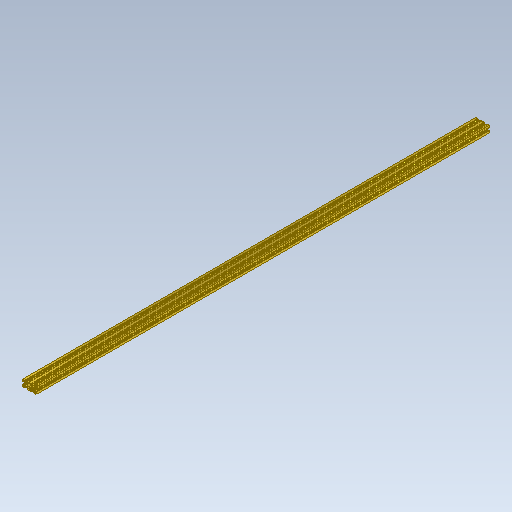
# Autodesk Inventor part: Perfil 30×60 6 rasgos_AST03006006
Saved by Autodesk Inventor 2025.2 (Build 292293000, 293)
## iProperties
Created: 2025-04-06
Part Number: Perfil 30×60 6 rasgos_AST03006006
Material: Ouro
Document SubType Name: Modeling
Designer: Gustavo Sousa
Density: 19.3 g/cm^3
Appearance: Metal quente 2400F
Author: Gustavo Sousa
Autodesk Inventor part; units mm, degrees
ref_plane "YZ Plane" through (0, 0, 0) normal (1, 0, 0) x (0, 1, 0)
ref_plane "XZ Plane" through (0, 0, 0) normal (0, 1, 0) x (-1, 0, 0)
ref_plane "XY Plane" through (0, 0, 0) normal (0, 0, 1) x (1, 0, 0)
sketch "Esboço1" plane through (0, 0, 0) normal (0, 0, 1) x (1, 0, 0)
  line L0 (-30, 15) -> (30, 15) construction
  circle A0 centre (-15, 0) radius 5 construction
  line L1 (-15, 0) -> (0, 15) construction
  line L2 (-22, 7) -> (-8, 7) construction
  line L3 (-19.1, 15) -> (-10.9, 15) construction
  line L4 (-30, 15) -> (-15, 15) construction
  line L5 (-22, 7) -> (-22, 0) construction
  line L6 (-30, 15) -> (-30, -15) construction
  line L7 (-19.1, 15) -> (-19.6, 15) construction
  line L8 (-19.6, 15) -> (-19.6, 14.5)
  line L9 (-19.6, 14.5) -> (-19.1, 14.5)
  line L10 (-19.1, 14.5) -> (-19.1, 15) construction
  line L11 (-19.1, 15) -> (-19.1, 12.8) construction
  line L12 (-19.1, 12.8) -> (-23.15, 12.8) construction
  line L13 (-19.1, 14.5) -> (-19.1, 12.8)
  line L14 (-22, 7) -> (-15, 0) construction
  line L15 (-22, 7) -> (-30, 15) construction
  arc A1 (-29.5, 15) -> (-30, 14.5) centre (-29.5, 14.5) ccw construction
  arc A2 (-29.5, 15) -> (-29.8536, 14.8536) centre (-29.5, 14.5) ccw
  line L16 (-29.5, 15) -> (-19.6, 15)
  line L17 (-23.15, 9.7056) -> (-20.4444, 7) construction
  line L18 (-23.15, 12.8) -> (-23.15, 9.7056) construction
  line L19 (-20.4444, 7) -> (-15, 7) construction
  circle A3 centre (-26.5, 11.5) radius 2.25 construction
  line L20 (-10.9, 15) -> (-10.4, 15) construction
  line L21 (-10.4, 15) -> (-10.4, 14.5)
  line L22 (-10.4, 14.5) -> (-10.9, 14.5)
  line L23 (-10.9, 14.5) -> (-10.9, 15) construction
  line L24 (-10.4, 15) -> (0, 15)
  line L25 (-10.9, 15) -> (-10.9, 12.8) construction
  line L26 (-10.9, 12.8) -> (-6.85, 12.8) construction
  line L27 (-10.9, 14.5) -> (-10.9, 12.8)
  line L28 (-9.5556, 7) -> (-6.85, 9.7056) construction
  line L29 (-6.85, 12.8) -> (-6.85, 9.7056) construction
  line L30 (-9.5556, 7) -> (-15, 7) construction
  line L31 (-8, 7) -> (-8, 0) construction
  line L32 (-22, 0) -> (-20, 0)
  line L33 (-10, 0) -> (-8, 0)
  line L34 (-4.65, 8.7944) -> (-8, 5.4444) construction
  arc A4 (-15, 5) -> (-20, 0) centre (-15, 0) ccw construction
  arc A5 (-10, 0) -> (-15, 5) centre (-15, 0) ccw
  line L35 (-4.65, 12.8) -> (0, 12.8) construction
  line L36 (0, 15) -> (0, 12.8) construction
  line L37 (-4.65, 12.8) -> (-4.65, 8.7944) construction
  line L38 (0, 15) -> (0, 12.8)
  line L39 (-8, 5.4444) -> (-8, 0) construction
  arc A6 (-24.909, 9.909) -> (-28.091, 13.091) centre (-26.5, 11.5) ccw
  arc A7 (-15, 5) -> (-18.5355, 3.5355) centre (-15, 0) ccw
  line L40 (-29.8536, 14.8536) -> (-18.5355, 3.5355)
  line L41 (-15, 5) -> (-15, 7)
  line L42 (-10, 0) -> (-8, 0)
  arc A8 (-20.5908, 7.1464) -> (-20.2373, 7) centre (-20.2373, 7.5) ccw
  arc A9 (-23.15, 9.9127) -> (-23.0036, 9.5592) centre (-22.65, 9.9127) ccw
  arc A10 (-22.65, 12.8) -> (-23.15, 12.3) centre (-22.65, 12.3) ccw
  line L43 (-22.65, 12.8) -> (-19.1, 12.8)
  line L44 (-23.15, 12.3) -> (-23.15, 9.9127)
  line L45 (-23.0036, 9.5592) -> (-20.5908, 7.1464)
  line L46 (-20.2373, 7) -> (-15, 7)
  arc A11 (-6.85, 12.3) -> (-7.35, 12.8) centre (-7.35, 12.3) ccw
  arc A12 (-6.9964, 9.5592) -> (-6.85, 9.9127) centre (-7.35, 9.9127) ccw
  arc A13 (-9.7627, 7) -> (-9.4092, 7.1464) centre (-9.7627, 7.5) ccw
  line L47 (-10.9, 12.8) -> (-7.35, 12.8)
  line L48 (-6.85, 12.3) -> (-6.85, 9.9127)
  line L49 (-6.9964, 9.5592) -> (-9.4092, 7.1464)
  line L50 (-9.7627, 7) -> (-15, 7)
  arc A14 (-7.8536, 5.5908) -> (-8, 5.2373) centre (-7.5, 5.2373) ccw
  arc A15 (-4.7964, 8.6479) -> (-4.65, 9.0015) centre (-5.15, 9.0015) ccw
  arc A16 (-4.15, 12.8) -> (-4.65, 12.3) centre (-4.15, 12.3) ccw
  line L51 (-8, 5.2373) -> (-8, 0)
  line L52 (-7.8536, 5.5908) -> (-4.7964, 8.6479)
  line L53 (-4.65, 9.0015) -> (-4.65, 12.3)
  line L54 (-4.15, 12.8) -> (0, 12.8)
  circle A17 centre (-18.5355, 3.5355) radius 1.1
  circle A18 centre (-11.4645, 3.5355) radius 1.1
  point P0 (0, 0)
  point P1 (-30, 0)
  point P2 (-10.9, 13.9)
  point P3 (-19.3134, 4.3134)
  point P4 (-17.6769, 4.2231)
  point P5 (-12.3231, 4.2231)
  point P6 (-10.7769, 2.6769)
  dimension "d0" = 15
  dimension "d1" = 60
  dimension "d3" = 15
  dimension "d4" = 10
  dimension "d6" = 8.2
  dimension "d7" = 15
  dimension "quadrado" = 0.5
  dimension "espessura" = 2.2
  dimension "d11" = 0.5
  dimension "d12" = 1.1
  dimension "d13" = 8
  dimension "d14" = 11.5
  dimension "d15" = 4.5
  dimension "d16" = 1.1
  dimension "d17" = 1.1
  dimension "d18" = 2
  dimension "d19" = 1.1
  dimension "d20" = 2.2
  dimension "d25" = 2.2
  dimension "d28" = 90
  constraints: 110 end point, 37 point on circle, 29 point on line, 24 tangent, 19 centre point, 17 collinear, 12 equal radius, 10 vertical, 9 horizontal, 7 parallel, 6 perpendicular, 5 coincident, 5 equal length, 5 horizontal alignment, 5 midpoint, 3 vertical alignment, 3 other
  measures "d0" distance from line of point (0, 0) L0
  measures "d1" distance of L0.start L0.end
  measures "d3" distance of point (0, 0) L1.start
  measures "d4" diameter of A0
  measures "d6" distance of L3.start L3.end
  measures "d7" distance of L0.start L4.end
  measures "quadrado" distance of L9.end L3.start
  measures "espessura" distance between parallel lines of L4 L12
  measures "d11" radius of A1
  measures "d12" distance between parallel lines of L15 L17
  measures "d13" distance of L4.end L19.end
  measures "d14" horizontal distance of L1.start A3.centre
  measures "d15" diameter of A3
  measures "d16" distance edge to line of A3 L18
  measures "d17" distance between parallel lines of L1 L28
  measures "d18" distance edge to line of A0 L5
  measures "d19" distance between parallel lines of L1 L34
  measures "d20" distance of L26.end L35.start
  measures "d25" diameter of A17
extrude "Extrusão1" add sketch "Esboço1" along normal mid plane 2000 contours L8 L9 L13 L43 A10 L44 A9 L45 A8 L46 L41 A7 A17 L40 A6 A2 L16
extrude "Extrusão2" add sketch "Esboço1" along normal mid plane 2000 contours L41 L50 A13 L49 A12 L48 A11 L47 L27 L22 L21 L24 L38 L54 A16 L53 A15 L52 A14 L51 L33 A5 A18
mirror "Espelhar1" about plane through (-29.8536, 14.8536, 0) normal (-0.7071068, -0.7071068, 0) of "Extrusão1"
mirror "Espelhar2" about plane through (0, 0, 0) normal (0, 1, 0) of "Extrusão1", "Espelhar1"
mirror "Espelhar3" about plane through (0, 0, 0) normal (0, 1, 0) of "Extrusão2"
mirror "Espelhar4" about plane through (0, 0, 0) normal (1, 0, 0) of "Extrusão1", "Extrusão2", "Espelhar1", "Espelhar2", "Espelhar3"
equation "\"d12\" = 0.5 * espessura"
equation "\"d16\" = 0.5 * espessura"
equation "\"d17\" = 0.5 * espessura"
equation "\"d19\" = 0.5 * espessura"
